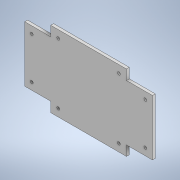
# Autodesk Inventor part: T960_and_RTK_mount
Saved by Autodesk Inventor 2020.2 (Build 242310000, 310)
## iProperties
Created: 2020-08-19
Part Number: T960_and_RTK_mount
Material: Generic
Document SubType Name: Modeling
Designer: Krishna Makhija
Density: 1 g/cm^3
Appearance: Default
Author: Krishna Makhija
Autodesk Inventor part; units mm, degrees
ref_plane "YZ Plane" through (0, 0, 0) normal (1, 0, 0) x (0, 1, 0)
ref_plane "XZ Plane" through (0, 0, 0) normal (0, 1, 0) x (-1, 0, 0)
ref_plane "XY Plane" through (0, 0, 0) normal (0, 0, 1) x (1, 0, 0)
sketch "Sketch2" plane through (0, 0, 0) normal (0, 1, 0) x (-1, 0, 0)
  circle A0 centre (-32, -32) radius 1.5001
  circle A1 centre (32, 32) radius 1.5001
  circle A2 centre (-32, 32) radius 1.5001
  circle A3 centre (32, -32) radius 1.5001
  circle A4 centre (60, 22) radius 1.5001
  circle A5 centre (60, -22) radius 1.5001
  circle A6 centre (-60, 22) radius 1.5001
  circle A7 centre (-60, -22) radius 1.5001
  line L0 (-67.4999, 29.5001) -> (67.4999, 29.5001)
  line L1 (67.4999, 29.5001) -> (67.4999, -29.5001)
  line L2 (67.4999, -29.5001) -> (-67.4999, -29.5001)
  line L3 (-67.4999, -29.5001) -> (-67.4999, 29.5001)
  line L4 (-67.4999, 29.5001) -> (67.4999, -29.5001) construction
  line L5 (67.4999, 29.5001) -> (-67.4999, -29.5001) construction
  line L6 (-40.0002, 40.0001) -> (40.0002, 40.0001)
  line L7 (40.0002, 40.0001) -> (40.0002, -40.0001)
  line L8 (40.0002, -40.0001) -> (-40.0002, -40.0001)
  line L9 (-40.0002, -40.0001) -> (-40.0002, 40.0001)
  line L10 (-40.0002, 40.0001) -> (40.0002, -40.0001) construction
  line L11 (40.0002, 40.0001) -> (-40.0002, -40.0001) construction
  point P0 (0, 0)
  point P1 (40.0002, 29.5001)
  point P2 (-40.0002, 29.5001)
  point P3 (-40.0002, -29.5001)
  point P4 (40.0002, -29.5001)
  constraints: 24 end point, 8 centre point, 4 parallel, 2 horizontal, 2 perpendicular
extrude "Extrusion1" add sketch "Sketch2" along normal blind 3
move or copy body "Move Body1" bodies to move or copy 1 copy no rotation origin (0, 0, 0) rotation axis (1, 0, 0) rotation angle 90 translate (0, 43.0001, 37.0001)
move or copy body "Move Body2" bodies to move or copy 1 copy no translate (10, 0, 0)
body "Solid1"
